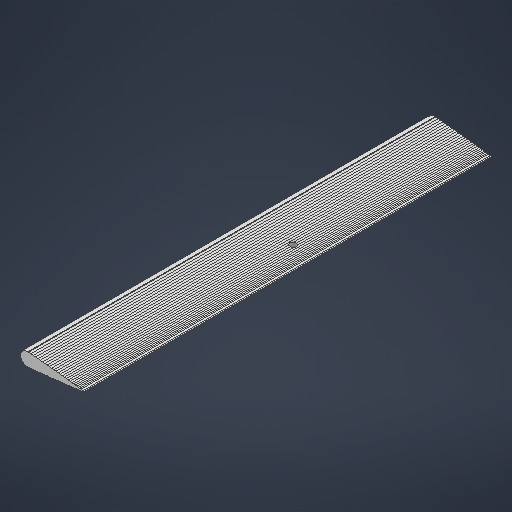
# Autodesk Inventor part: horizontal_stab_elevator
Saved by Autodesk Inventor 2026 (Build 300175050, 175E)
## iProperties
Created: 2026-02-21
Part Number: horizontal_stab_elevator
Material: Všeobecné
Document SubType Name: Modeling
Designer: marti
Density: 1 g/cm^3
Appearance: Výchozí
Author: marti
Autodesk Inventor part; units mm, degrees
ref_plane "YZ Plane" through (0, 0, 0) normal (1, 0, 0) x (0, 1, 0)
ref_plane "XZ Plane" through (0, 0, 0) normal (0, 1, 0) x (-1, 0, 0)
ref_plane "XY Plane" through (0, 0, 0) normal (0, 0, 1) x (1, 0, 0)
sketch "Náčrt1" plane through (0, 0, 0) normal (0, 0, 1) x (1, 0, 0)
  line L0 (52.3561, -3.2889) -> (52.7026, -3.258)
  line L1 (52.7026, -3.258) -> (53.8641, -3.1519)
  line L2 (53.8641, -3.1519) -> (55.0221, -3.0436)
  line L3 (55.0221, -3.0436) -> (56.1757, -2.9334)
  line L4 (56.1757, -2.9334) -> (57.324, -2.8213)
  line L5 (57.324, -2.8213) -> (58.466, -2.7076)
  line L6 (58.466, -2.7076) -> (59.6005, -2.5924)
  line L7 (59.6005, -2.5924) -> (60.7266, -2.476)
  line L8 (60.7266, -2.476) -> (61.843, -2.3584)
  line L9 (61.843, -2.3584) -> (62.9485, -2.2399)
  line L10 (62.9485, -2.2399) -> (64.0421, -2.1207)
  line L11 (64.0421, -2.1207) -> (65.124, -2.0008)
  line L12 (65.124, -2.0008) -> (66.1891, -1.8799)
  line L13 (66.1891, -1.8799) -> (67.2379, -1.7589)
  line L14 (67.2379, -1.7589) -> (68.2689, -1.6383)
  line L15 (68.2689, -1.6383) -> (69.2801, -1.5181)
  line L16 (69.2801, -1.5181) -> (70.27, -1.3988)
  line L17 (70.27, -1.3988) -> (71.2363, -1.2806)
  line L18 (71.2363, -1.2806) -> (72.1771, -1.164)
  line L19 (72.1771, -1.164) -> (73.0899, -1.0493)
  line L20 (73.0899, -1.0493) -> (73.972, -0.937)
  line L21 (73.972, -0.937) -> (74.8205, -0.8276)
  line L22 (74.8205, -0.8276) -> (75.6321, -0.7216)
  line L23 (75.6321, -0.7216) -> (76.4028, -0.6198)
  line L24 (76.4028, -0.6198) -> (77.1281, -0.5229)
  line L25 (77.1281, -0.5229) -> (77.8025, -0.4319)
  line L26 (77.8025, -0.4319) -> (78.4188, -0.3479)
  line L27 (78.4188, -0.3479) -> (78.9642, -0.245)
  line L28 (78.9642, -0.245) -> (79.4284, -0.1574)
  line L29 (79.4284, -0.1574) -> (79.7982, -0.1291)
  line L30 (79.7982, -0.1291) -> (80, -0.1136)
  line L31 (52.3786, 3.287) -> (52.7026, 3.2581)
  line L32 (52.7026, 3.2581) -> (53.864, 3.152)
  line L33 (53.864, 3.152) -> (55.022, 3.0437)
  line L34 (55.022, 3.0437) -> (56.1756, 2.9335)
  line L35 (56.1756, 2.9335) -> (57.3239, 2.8214)
  line L36 (57.3239, 2.8214) -> (58.4658, 2.7077)
  line L37 (58.4658, 2.7077) -> (59.6004, 2.5925)
  line L38 (59.6004, 2.5925) -> (60.7264, 2.4761)
  line L39 (60.7264, 2.4761) -> (61.843, 2.3585)
  line L40 (61.843, 2.3585) -> (62.9486, 2.24)
  line L41 (62.9486, 2.24) -> (64.0421, 2.1208)
  line L42 (64.0421, 2.1208) -> (65.124, 2.0009)
  line L43 (65.124, 2.0009) -> (66.1891, 1.88)
  line L44 (66.1891, 1.88) -> (67.238, 1.759)
  line L45 (67.238, 1.759) -> (68.2689, 1.6383)
  line L46 (68.2689, 1.6383) -> (69.2801, 1.5182)
  line L47 (69.2801, 1.5182) -> (70.27, 1.3989)
  line L48 (70.27, 1.3989) -> (71.2364, 1.2807)
  line L49 (71.2364, 1.2807) -> (72.1771, 1.1641)
  line L50 (72.1771, 1.1641) -> (73.0899, 1.0494)
  line L51 (73.0899, 1.0494) -> (73.972, 0.937)
  line L52 (73.972, 0.937) -> (74.8205, 0.8276)
  line L53 (74.8205, 0.8276) -> (75.6321, 0.7217)
  line L54 (75.6321, 0.7217) -> (76.4028, 0.6199)
  line L55 (76.4028, 0.6199) -> (77.1281, 0.523)
  line L56 (77.1281, 0.523) -> (77.8025, 0.432)
  line L57 (77.8025, 0.432) -> (78.4188, 0.348)
  line L58 (78.4188, 0.348) -> (78.9679, 0.2725)
  line L59 (78.9679, 0.2725) -> (79.4365, 0.208)
  line L60 (79.4365, 0.208) -> (79.8021, 0.1566)
  line L61 (79.8021, 0.1566) -> (80, 0.1287)
  line L62 (80, 0.1287) -> (80, -0.1136)
  line L63 (49.176, -1.5573) -> (50.2021, -1.4704)
  line L64 (50.2021, -1.4704) -> (51.3632, -1.3695)
  line L65 (51.3632, -1.3695) -> (52.5228, -1.2661)
  line L66 (52.5228, -1.2661) -> (53.68, -1.1604)
  line L67 (53.68, -1.1604) -> (54.8339, -1.0525)
  line L68 (54.8339, -1.0525) -> (55.9835, -0.9426)
  line L69 (55.9835, -0.9426) -> (57.1278, -0.831)
  line L70 (57.1278, -0.831) -> (58.2659, -0.7176)
  line L71 (58.2659, -0.7176) -> (59.3966, -0.6029)
  line L72 (59.3966, -0.6029) -> (60.519, -0.4868)
  line L73 (60.519, -0.4868) -> (61.6317, -0.3696)
  line L74 (61.6317, -0.3696) -> (62.7336, -0.2515)
  line L75 (62.7336, -0.2515) -> (63.8236, -0.1327)
  line L76 (63.8236, -0.1327) -> (65.0211, 0)
  line L77 (65.0211, 0) -> (63.8236, 0.1327)
  line L78 (63.8236, 0.1327) -> (62.7337, 0.2516)
  line L79 (62.7337, 0.2516) -> (61.6317, 0.3697)
  line L80 (61.6317, 0.3697) -> (60.5188, 0.4869)
  line L81 (60.5188, 0.4869) -> (59.3965, 0.6029)
  line L82 (59.3965, 0.6029) -> (58.2657, 0.7177)
  line L83 (58.2657, 0.7177) -> (57.1277, 0.831)
  line L84 (57.1277, 0.831) -> (55.9833, 0.9427)
  line L85 (55.9833, 0.9427) -> (54.8338, 1.0526)
  line L86 (54.8338, 1.0526) -> (53.6799, 1.1604)
  line L87 (53.6799, 1.1604) -> (52.5228, 1.2662)
  line L88 (52.5228, 1.2662) -> (51.3632, 1.3696)
  line L89 (51.3632, 1.3696) -> (50.2021, 1.4705)
  line L90 (50.2021, 1.4705) -> (49.0403, 1.5688)
  arc A0 (52.3786, 3.287) -> (52.401, -3.2849) centre (52.0854, 0) ccw
  dimension "d10" = 3.3
  constraints: 182 end point, 4 point on circle, 2 collinear, 1 centre point, 1 point on line, 1 tangent, 1 vertical, 21 other
  measures "d10" radius of A0
extrude "Vysunutí1" add sketch "Náčrt1" along normal mid plane 200
sketch "Náčrt2" plane through (76.4028, 0.6199, 100) normal (0.1324, 0.9912, 0) x (0.9912, -0.1324, 0)
  circle A0 centre (-6.3695, 112.5) radius 1.5
  line L0 (3.6305, 200) -> (3.6305, 0) projected
  circle A1 centre (-6.3695, 112.5) radius 5
  point P0 (-75.6482, 100)
  point P1 (3.6305, 100)
  dimension "d14" = 3
  dimension "d15" = 12.5
  dimension "d17" = 10
  dimension "d23" = 10
  constraints: 2 centre point, 1 coincident, 1 midpoint
  measures "d14" diameter of A0
  measures "d15" vertical distance of point (3.63, 100) A0.centre
  measures "d17" distance from line of L0 A0.centre
  measures "d23" diameter of A1
extrude "Vysunutí6" cut sketch "Náčrt2" along normal through all both and the other way through all contours A0
sketch "Náčrt4" plane through (0, 0, 100) normal (0, 0, 1) x (1, 0, 0)
  arc A0 (52.3786, 3.287) -> (52.3561, -3.2889) centre (52.0854, 0) ccw projected
  circle A1 centre (52.0854, 0) radius 2
  circle A2 centre (57.0854, 0) radius 1.5
  point P0 (0, 0)
  dimension "d31" = 4
  dimension "d32" = 3
  dimension "d33" = 5
  constraints: 2 centre point, 1 coincident
  measures "d31" diameter of A1
  measures "d32" diameter of A2
  measures "d33" distance of A2.centre A0.centre
extrude "Vysunutí7" [suppressed]
